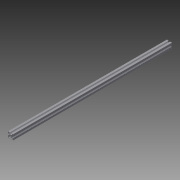
# Autodesk Inventor part: 600 beam
Saved by Autodesk Inventor 2015 (Build 190159000, 159)
## iProperties
Created: 2015-01-27
Part Number: 600 beam
Material: Generic
Document SubType Name: Modeling
Designer: Joseph
Density: 1 g/cm^3
Appearance: Aluminum - Dark
Author: Joseph
Autodesk Inventor part; units mm, degrees
ref_plane "YZ Plane" through (0, 0, 0) normal (1, 0, 0) x (0, 1, 0)
ref_plane "XZ Plane" through (0, 0, 0) normal (0, 1, 0) x (-1, 0, 0)
ref_plane "XY Plane" through (0, 0, 0) normal (0, 0, 1) x (1, 0, 0)
sketch "Sketch1" plane through (0, 0, 0) normal (0, 0, 1) x (1, 0, 0)
  circle A0 centre (0, 0) radius 2.5
  line L0 (2.9774, 3.8259) -> (-2.9774, 3.8259)
  line L1 (-3.8259, 2.9774) -> (-3.8259, -2.9774)
  line L2 (-3.8259, -2.9774) -> (-8.8, -7.9515)
  line L3 (-7.9515, -8.8) -> (-2.9774, -3.8259)
  line L4 (2.9774, -3.8259) -> (7.9515, -8.8)
  line L5 (3.8259, 2.9774) -> (8.8, 7.9515)
  line L6 (8.8, -7.9515) -> (3.8259, -2.9774)
  line L7 (7.9515, 8.8) -> (2.9774, 3.8259)
  line L8 (-2.9774, 3.8259) -> (-7.9515, 8.8)
  line L9 (-8.8, 7.9515) -> (-3.8259, 2.9774)
  line L10 (-2.9774, -3.8259) -> (2.9774, -3.8259)
  line L11 (3.8259, -2.9774) -> (3.8259, 2.9774)
  line L12 (-3.1451, -8.8) -> (-2.6278, -10)
  line L13 (-3.1451, -8.8) -> (-7.9515, -8.8)
  line L14 (-10, -10) -> (-2.6278, -10)
  line L15 (2.6278, -10) -> (10, -10)
  line L16 (7.9515, -8.8) -> (3.1451, -8.7999)
  circle A1 centre (0, 0) radius 3.8259 construction
  line L17 (0, 0) -> (7.0677, 7.0677) construction
  circle A2 centre (2.7053, 2.7053) radius 1.1531 construction
  line L18 (-13.2321, 0) -> (16.76, 0) construction
  circle A3 centre (0, 0) radius 4.848 construction
  line L19 (2.6278, -10) -> (3.1451, -8.7999)
  line L20 (-8.8, -7.9515) -> (-8.8, -3.1451)
  line L21 (-8.8, -3.1451) -> (-10, -2.6278)
  line L22 (-8.8, 7.9515) -> (-8.8, 3.1451)
  line L23 (-8.8, 3.1451) -> (-10, 2.6278)
  line L24 (-7.9515, 8.8) -> (-3.1451, 8.8)
  line L25 (-3.1451, 8.8) -> (-2.6278, 10)
  line L26 (7.9515, 8.8) -> (3.1451, 8.8)
  line L27 (3.1451, 8.8) -> (2.6278, 10)
  line L28 (8.8, 7.9515) -> (8.8, 3.1451)
  line L29 (8.8, 3.1451) -> (10, 2.6278)
  line L30 (8.8, -7.9515) -> (8.8, -3.1451)
  line L31 (8.8, -3.1451) -> (10, -2.6278)
  line L32 (-10, 10) -> (-10, 2.6278)
  line L33 (-10, -2.6278) -> (-10, -10)
  line L34 (10, 10) -> (2.6278, 10)
  line L35 (-2.6278, 10) -> (-10, 10)
  line L36 (10, -10) -> (10, -2.6278)
  line L37 (10, 2.6278) -> (10, 10)
  point P0 (3.8259, 0)
  point P1 (-0.0241, 0)
  point P2 (-3.8259, 0)
  dimension "d0" = 20
  dimension "d1" = 20
  dimension "d2" = 5
  dimension "d3" = 1.2
  dimension "d4" = 1.2
  dimension "d5" = 1.2
  dimension "d6" = 1.2
  dimension "d7" = 20
  dimension "d8" = 1.2
  dimension "d9" = 1.2
  dimension "d10" = 1.2
  dimension "d11" = 1.2
  dimension "d12" = 1.2
  dimension "d13" = 20
  constraints: 77 end point, 23 equal length, 17 parallel, 9 horizontal, 7 point on circle, 6 perpendicular, 5 vertical, 3 centre point, 3 coincident, 2 horizontal alignment, 2 midpoint, 2 point on line, 3 other
  measures "d0" distance of L32.start L34.start
  measures "d1" distance of L34.start L15.end
  measures "d2" diameter of A0
  measures "d3" distance of L7.start L5.end
  measures "d4" distance between parallel lines of L6 L4
  measures "d5" distance between parallel lines of L8 L9
  measures "d6" distance between parallel lines of L2 L3
  measures "d7" distance of L32.start L14.start
  measures "d8" distance between parallel lines of L35 L24
  measures "d9" distance between parallel lines of L32 L22
  measures "d10" distance between parallel lines of L20 L33
  measures "d11" distance between parallel lines of L34 L26
  measures "d12" distance between parallel lines of L37 L28
  measures "d13" distance between parallel lines of L36 L33
extrude "Extrusion1" add sketch "Sketch1" along normal blind 600
fillet "Fillet1" radius 0.5 12 edges at (-10, 10, 300) (-7.9515, 8.8, 300) (-8.8, 7.9515, 300) (-10, -10, 300) (-7.9515, -8.8, 300) (-8.8, -7.9515, 300) (10, -10, 300) (7.9515, -8.8, 300) (8.8, -7.9515, 300) (7.9515, 8.8, 300) (10, 10, 300) (8.8, 7.9515, 300)
body "Solid1"
